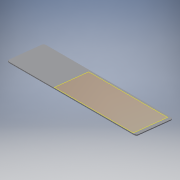
# Autodesk Inventor part: Baseplate
Saved by Autodesk Inventor 2016 (Build 200138000, 138)
## iProperties
Created: 2021-01-31
Part Number: Baseplate
Material: Generic
Document SubType Name: Modeling
Designer: Tom
Density: 1 g/cm^3
Appearance: Default
Author: Tom
Autodesk Inventor part; units mm, degrees
ref_plane "YZ Plane" through (0, 0, 0) normal (1, 0, 0) x (0, 1, 0)
ref_plane "XZ Plane" through (0, 0, 0) normal (0, 1, 0) x (-1, 0, 0)
ref_plane "XY Plane" through (0, 0, 0) normal (0, 0, 1) x (1, 0, 0)
ref_plane "Work Plane1" through (134.3476, -19.5515, -187.1593) normal (0, 0.1061113, 0.9943543) x (-1, 0, 0)
sketch "Sketch1" plane through (134.3476, -19.5515, -187.1593) normal (0, 0.1061113, 0.9943543) x (-1, 0, 0)
  line L0 (-256.9788, 108.2703) -> (-256.9788, -5.086)
  ellipse E0 centre (-252.2288, 108.2703) end of major axis (-256.9788, 108.2703) minor radius 4.7232 (-252.2288, 112.9935) -> (-256.9788, 108.2703) ccw
  line L1 (180.0212, 112.9935) -> (-252.2288, 112.9935)
  ellipse E1 centre (180.0212, 108.2703) end of major axis (175.2712, 108.2703) minor radius 4.7232 (184.7712, 108.2703) -> (180.0212, 112.9935) ccw
  line L2 (184.7712, -5.086) -> (184.7712, 108.2703)
  line L3 (-252.2288, -9.8092) -> (180.0212, -9.8092)
  ellipse E2 centre (-252.2288, -5.086) end of major axis (-256.9788, -5.086) minor radius 4.7232 (-256.9788, -5.086) -> (-252.2288, -9.8092) ccw
  line L4 (187.7712, -5.086) -> (187.7712, 108.2703)
  line L5 (180.0212, 115.9935) -> (-252.2288, 115.9935)
  line L6 (-259.9788, 108.2703) -> (-259.9788, -5.086)
  line L7 (-252.2288, -12.8092) -> (180.0212, -12.8092)
  arc A0 (180.0212, -9.8092) -> (184.7712, -5.086) centre (180.0212, -5.0592) ccw
  arc A1 (180.0212, -12.8092) -> (187.7712, -5.086) centre (180.0212, -5.0592) ccw
  spline S0 degree 5 poles (187.7712, 108.2703) (187.7712, 109.486) (187.5312, 110.7016) (187.051, 111.854) (185.6639, 113.906) (183.6042, 115.2817) (182.451, 115.7563) (181.2361, 115.9935) (180.0212, 115.9935) knots 0 0 0 0 0 0 0.500147 0.500147 0.500147 1 1 1 1 1 1
  spline S1 degree 5 poles (-252.2288, 115.9935) (-253.4437, 115.9935) (-254.6586, 115.7563) (-255.8118, 115.2817) (-257.8715, 113.906) (-259.2586, 111.854) (-259.7388, 110.7016) (-259.9788, 109.486) (-259.9788, 108.2703) knots 0 0 0 0 0 0 0.499853 0.499853 0.499853 1 1 1 1 1 1
  spline S2 degree 5 poles (-259.9788, -5.086) (-259.9788, -6.3017) (-259.7388, -7.5173) (-259.2586, -8.6697) (-257.8715, -10.7217) (-255.8118, -12.0974) (-254.6586, -12.572) (-253.4437, -12.8092) (-252.2288, -12.8092) knots 0 0 0 0 0 0 0.500147 0.500147 0.500147 1 1 1 1 1 1
  constraints: 16 end point, 4 point on circle, 2 centre point, 21 other
extrude "Extrusion1" add sketch "Sketch1" against normal blind 3 contours E0 L1 E1 L2 A0 L3 E2 L0 | A1 L7 S2 L6 S1 L5 S0 L4
body "Solid1"
